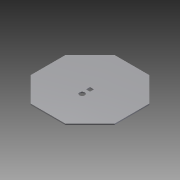
# Autodesk Inventor part: Robot-Upper-Base
Saved by Autodesk Inventor 2012 (Build 160160000, 160)
## iProperties
Created: 2013-07-14
Part Number: Robot-Upper-Base
Material: Default
Document SubType Name: Modeling
Designer: joe_000
Density: 1 g/cm^3
Author: joe_000
Autodesk Inventor part; units mm, degrees
ref_plane "YZ Plane" through (0, 0, 0) normal (1, 0, 0) x (0, 1, 0)
ref_plane "XZ Plane" through (0, 0, 0) normal (0, 1, 0) x (-1, 0, 0)
ref_plane "XY Plane" through (0, 0, 0) normal (0, 0, 1) x (1, 0, 0)
sketch "Sketch1" plane through (0, 0, 0) normal (0, 1, 0) x (-1, 0, 0)
  line L0 (-203.2, 84.1682) -> (-84.1682, 203.2)
  line L1 (-84.1682, 203.2) -> (84.1682, 203.2)
  line L2 (84.1682, 203.2) -> (203.2, 84.1682)
  line L3 (203.2, 84.1682) -> (203.2, -84.1682)
  line L4 (203.2, -84.1682) -> (84.1682, -203.2)
  line L5 (84.1682, -203.2) -> (-84.1682, -203.2)
  line L6 (-84.1682, -203.2) -> (-203.2, -84.1682)
  line L7 (-203.2, -84.1682) -> (-203.2, 84.1682)
  point P0 (0, 0)
  point P1 (0, 0)
  dimension "d0" = 406.4
  constraints: 16 end point, 1 coincident, 1 vertical, 17 other
  measures "d0" distance between parallel lines of L7 L3
extrude "Extrusion1" add sketch "Sketch1" along normal blind 5.5563
sketch "Sketch2" plane through (0, 5.5563, 0) normal (0, 1, 0) x (1, 0, 0)
  line L0 (9.525, -9.525) -> (-9.525, -9.525)
  line L1 (-9.525, -9.525) -> (-9.525, 9.525)
  line L2 (-9.525, 9.525) -> (9.525, 9.525)
  line L3 (9.525, 9.525) -> (9.525, -9.525)
  circle A0 centre (0, -38.1) radius 12.7
  point P0 (0, 0)
  dimension "d3" = 19.05
  dimension "d4" = 19.05
  dimension "d5" = 9.525
  dimension "d6" = 9.525
  dimension "d9" = 25.4
  dimension "d10" = 38.1
  constraints: 8 end point, 2 parallel, 1 centre point, 1 horizontal, 1 perpendicular
  measures "d3" distance of L1.end L2.end
  measures "d4" distance of L0.end L1.end
  measures "d5" distance from line of point (0, 0) L0
  measures "d6" distance from line of point (0, 0) L3
  measures "d9" diameter of A0
  measures "d10" distance of point (0, 0) A0.centre
extrude "Extrusion2" cut sketch "Sketch2" against normal through all
equation "\"d0\" = BaseWidth"
equation "\"d3\" = MastWidth"
equation "\"d4\" = d3"
equation "\"d5\" = 0.5 * d3"
equation "\"d6\" = 0.5 * d3"
equation "\"d9\" = WireHoleDiameter"
equation "\"d10\" = WireHoleOffset"
equation "\"BaseWidth\" = 406.4"
equation "\"MastWidth\" = 19.05"
equation "\"WireHoleDiameter\" = 25.4"
equation "\"WireHoleOffset\" = 38.1"
body "Solid1"
